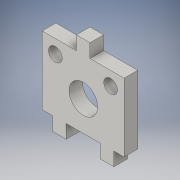
# Autodesk Inventor part: Near Holder
Saved by Autodesk Inventor 2016 (Build 200138000, 138)
## iProperties
Created: 2016-04-25
Part Number: Near Holder
Material: PVC-Piping
Document SubType Name: Modeling
Designer: rubenjm
Density: 1.4 g/cm^3
Appearance: Smooth - White
Author: rubenjm
Autodesk Inventor part; units mm, degrees
ref_plane "YZ Plane" through (0, 0, 0) normal (1, 0, 0) x (0, 1, 0)
ref_plane "XZ Plane" through (0, 0, 0) normal (0, 1, 0) x (-1, 0, 0)
ref_plane "XY Plane" through (0, 0, 0) normal (0, 0, 1) x (1, 0, 0)
sketch "Sketch1" plane through (0, 0, 0) normal (0, 0, 1) x (1, 0, 0)
  circle A0 centre (44.45, 27.9405) radius 6.985 construction
  circle A1 centre (18.5683, 50.8) radius 6.35 construction
  line L0 (6.35, 63.5) -> (6.35, 50.8) construction
  line L1 (6.35, 50.8) -> (19.05, 50.8) construction
  line L2 (19.05, 50.8) -> (19.05, 63.5) construction
  line L3 (19.05, 63.5) -> (6.35, 63.5) construction
  circle A2 centre (70.0106, 50.8) radius 6.35 construction
  line L4 (31.779, 27.94) -> (38.1948, 39.0525) construction
  line L5 (38.1948, 39.0525) -> (51.0264, 39.0525) construction
  line L6 (51.0264, 39.0525) -> (57.4422, 27.94) construction
  line L7 (57.4422, 27.94) -> (51.0264, 16.8275) construction
  line L8 (51.0264, 16.8275) -> (38.1948, 16.8275) construction
  line L9 (6.35, 63.5) -> (6.35, 0)
  line L10 (82.55, 0) -> (82.55, 63.5)
  line L11 (82.55, 63.5) -> (6.35, 63.5)
  line L12 (31.779, 27.94) -> (38.1948, 16.8275) construction
  line L13 (44.45, 0) -> (44.45, 27.9405) construction
  line L14 (44.45, 27.9405) -> (44.45, 63.5) construction
  line L15 (44.45, 0) -> (60.325, 0)
  line L16 (44.45, 0) -> (60.325, 0)
  line L17 (73.025, 0) -> (73.025, -12.7)
  line L18 (73.025, -12.7) -> (60.325, -12.7)
  line L19 (60.325, -12.7) -> (60.325, 0)
  line L20 (73.025, 0) -> (82.55, 0)
  line L21 (44.45, 0) -> (28.575, 0)
  line L22 (44.45, 0) -> (28.575, 0)
  line L23 (15.875, 0) -> (15.875, -12.7)
  line L24 (15.875, -12.7) -> (28.575, -12.7)
  line L25 (28.575, -12.7) -> (28.575, 0)
  line L26 (15.875, 0) -> (6.35, 0)
  point P0 (0, 0)
  point P1 (0, 0)
  point P2 (12.8606, 0)
  dimension "d0" = 76.2
  dimension "d1" = 63.5
  dimension "d21" = 15.875
  dimension "d22" = 0
  dimension "d24" = 12.7
  dimension "d25" = 12.7
  constraints: 54 end point, 5 symmetric about line, 4 parallel, 3 centre point, 2 horizontal, 1 collinear, 1 midpoint, 1 perpendicular, 1 point on line
  measures "d0" distance of L10.end L0.start
  measures "d1" distance of L10.start L10.end
  measures "d21" distance of L13.start L15.end
  measures "d22" distance between parallel lines of L15 L16
  measures "d24" distance of L17.end L18.end
  measures "d25" distance of L17.start L17.end
extrude "Extrusion1" add sketch "Sketch1" along normal blind 12.7
sketch "Sketch2" plane through (0, 0, 12.7) normal (0, 0, 1) x (1, 0, 0)
  circle A0 centre (18.5683, 50.8) radius 6.35
  line L0 (31.779, 27.94) -> (38.1948, 39.0525) construction
  line L1 (44.45, 0) -> (44.45, 15.875) construction
  line L2 (38.1948, 39.0525) -> (51.0264, 39.0525) construction
  line L3 (51.0264, 16.8275) -> (38.1948, 16.8275) construction
  circle A1 centre (44.6106, 27.94) radius 13.335
  line L4 (51.0264, 39.0525) -> (57.4422, 27.94) construction
  line L5 (57.4422, 27.94) -> (51.0264, 16.8275) construction
  circle A2 centre (70.0106, 50.8) radius 6.35
  line L6 (44.45, 0) -> (44.45, 27.94) construction
  line L7 (31.779, 27.94) -> (38.1948, 16.8275) construction
  line L8 (44.45, 0) -> (44.45, 27.94) construction
  line L9 (6.35, 63.5) -> (82.55, 63.5) construction
  line L10 (44.45, 27.94) -> (44.45, 63.5) construction
  line L11 (82.55, 63.5) -> (6.35, 63.5) construction
  dimension "d8" = 26.67
  dimension "d9" = 12.7
  dimension "d10" = 12.7
  dimension "d17" = 27.94
  constraints: 22 end point, 3 centre point, 1 collinear, 1 horizontal, 1 midpoint, 1 point on line
  measures "d8" diameter of A1
  measures "d9" diameter of A0
  measures "d10" diameter of A2
  measures "d17" vertical distance of L1.start A1.centre
extrude "Extrusion2" cut sketch "Sketch2" against normal blind 12.7
sketch "Sketch3" plane through (0, 0, 12.7) normal (0, 0, 1) x (1, 0, 0)
  line L0 (28.575, 0) -> (60.325, 0) construction
  line L1 (44.45, 0) -> (44.45, 63.5) construction
  line L2 (82.55, 63.5) -> (6.35, 63.5) construction
  line L3 (44.45, 63.5) -> (44.45, 69.85) construction
  line L4 (38.1, 76.2) -> (50.8, 76.2)
  line L5 (50.8, 76.2) -> (50.8, 63.5)
  line L6 (50.8, 63.5) -> (38.1, 63.5)
  line L7 (38.1, 63.5) -> (38.1, 76.2)
  line L8 (38.1, 76.2) -> (50.8, 63.5) construction
  line L9 (50.8, 76.2) -> (38.1, 63.5) construction
  point P0 (0, 0)
  dimension "d26" = 6.35
  dimension "d27" = 12.7
  dimension "d28" = 12.7
  constraints: 16 end point, 4 midpoint, 2 parallel, 1 horizontal, 1 perpendicular, 1 point on line
  measures "d26" distance of L1.end L3.end
  measures "d27" distance of L5.end L6.end
  measures "d28" distance of L4.end L5.end
extrude "Extrusion3" add sketch "Sketch3" against normal blind 12.7
body "Solid1"
